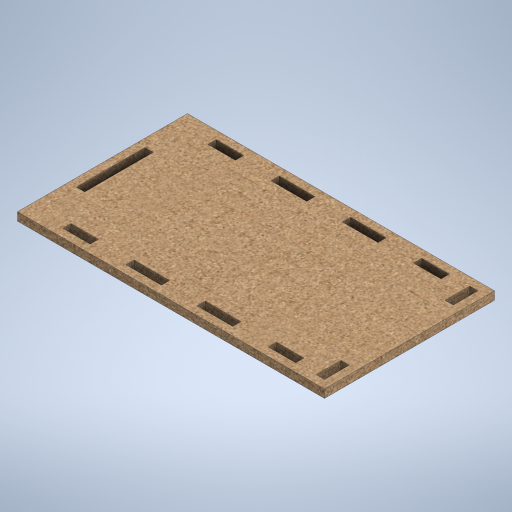
# Autodesk Inventor part: Case_Base1
Saved by Autodesk Inventor 2024 (Build 280153000, 153)
## iProperties
Created: 2023-11-23
Part Number: Case_Base1
Material: MDF Tablero de fibras de densidad media
Document SubType Name: Modeling
Designer: marco
Density: 0.8 g/cm^3
Appearance: Cartón - Ondulado
Author: marco
Autodesk Inventor part; units mm, degrees
ref_plane "YZ Plane" through (0, 0, 0) normal (1, 0, 0) x (0, 1, 0)
ref_plane "XZ Plane" through (0, 0, 0) normal (0, 1, 0) x (-1, 0, 0)
ref_plane "XY Plane" through (0, 0, 0) normal (0, 0, 1) x (1, 0, 0)
sketch "Boceto1" plane through (0, 0, 0) normal (0, 1, 0) x (-1, 0, 0)
  line L0 (-53, -19) -> (-53, -28)
  line L1 (-50, -19) -> (-50, -28)
  line L2 (32.5, -28) -> (32.5, -25)
  line L3 (42.5, -28) -> (32.5, -28)
  line L4 (42.5, -25) -> (42.5, -28)
  line L5 (50, -12.5) -> (50, 12.5)
  line L6 (53, -12.5) -> (50, -12.5)
  line L7 (53, 12.5) -> (53, -12.5)
  line L8 (50, 12.5) -> (53, 12.5)
  line L9 (-53, 28) -> (-50, 28)
  line L10 (-53, 19) -> (-53, 28)
  line L11 (-50, 19) -> (-53, 19)
  line L12 (-50, 28) -> (-50, 19)
  line L13 (-50, -19) -> (-53, -19)
  line L14 (-53, -28) -> (-50, -28)
  line L15 (-19.5, 28) -> (-6.5, 28)
  line L16 (-19.5, 25) -> (-19.5, 28)
  line L17 (-6.5, 25) -> (-19.5, 25)
  line L18 (-6.5, 28) -> (-6.5, 25)
  line L19 (6.5, 28) -> (19.5, 28)
  line L20 (6.5, 25) -> (6.5, 28)
  line L21 (19.5, 25) -> (6.5, 25)
  line L22 (19.5, 28) -> (19.5, 25)
  line L23 (-6.5, -25) -> (-6.5, -28)
  line L24 (-19.5, -25) -> (-6.5, -25)
  line L25 (-19.5, -28) -> (-19.5, -25)
  line L26 (-6.5, -28) -> (-19.5, -28)
  line L27 (19.5, -25) -> (19.5, -28)
  line L28 (6.5, -25) -> (19.5, -25)
  line L29 (6.5, -28) -> (6.5, -25)
  line L30 (19.5, -28) -> (6.5, -28)
  line L31 (-42.5, 28) -> (-42.5, 25)
  line L32 (-32.5, 28) -> (-42.5, 28)
  line L33 (-32.5, 25) -> (-32.5, 28)
  line L34 (-42.5, 25) -> (-32.5, 25)
  line L35 (42.5, -28) -> (42.5, -25)
  line L36 (32.5, -28) -> (42.5, -28)
  line L37 (32.5, -25) -> (32.5, -28)
  line L38 (42.5, -25) -> (32.5, -25)
  line L39 (42.5, -25) -> (32.5, -25)
  line L40 (42.5, -28) -> (42.5, -25)
  line L41 (32.5, -28) -> (42.5, -28)
  line L42 (32.5, -25) -> (32.5, -28)
  line L43 (42.5, 25) -> (32.5, 25)
  line L44 (42.5, 28) -> (42.5, 25)
  line L45 (32.5, 28) -> (42.5, 28)
  line L46 (32.5, 25) -> (32.5, 28)
  line L47 (-56, 31) -> (-56, -31)
  line L48 (56, 31) -> (-56, 31)
  line L49 (56, -31) -> (56, 31)
  line L50 (-56, -31) -> (56, -31)
  line L51 (-32.5, -28) -> (-32.5, -25)
  line L52 (-42.5, -28) -> (-32.5, -28)
  line L53 (-42.5, -25) -> (-42.5, -28)
  line L54 (-32.5, -25) -> (-42.5, -25)
  point P0 (0, 0)
  constraints: 110 end point
extrude "Extrusión1" add sketch "Boceto1" along normal blind 3
